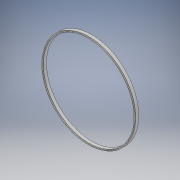
# Autodesk Inventor part: 뚜겅
Saved by Autodesk Inventor 2019.5 (Build 235369000, 369)
## iProperties
Created: 2021-07-28
Part Number: 뚜겅
Material: 일반
Document SubType Name: Modeling
Designer: msj19
Density: 1 g/cm^3
Appearance: 기본값
Author: msj19
Autodesk Inventor part; units mm, degrees
ref_plane "우측면도" through (0, 0, 0) normal (1, 0, 0) x (0, 1, 0)
ref_plane "평면도" through (0, 0, 0) normal (0, 1, 0) x (-1, 0, 0)
ref_plane "정면도" through (0, 0, 0) normal (0, 0, 1) x (1, 0, 0)
sketch "스케치1" plane through (0, 0, 0) normal (0, 0, 1) x (1, 0, 0)
  circle A0 centre (0, 0) radius 10
  circle A1 centre (0, 0) radius 155
  circle A2 centre (0, 0) radius 150
  line L0 (-100, -100) -> (100, -100)
  line L1 (100, -100) -> (100, 100)
  line L2 (100, 100) -> (-100, 100)
  line L3 (-100, 100) -> (-100, -100)
  line L4 (-100, -100) -> (100, 100) construction
  line L5 (100, -100) -> (-100, 100) construction
  point P0 (-92, -32.0118)
  dimension "d0" = 5
  dimension "d9" = 97.4103
  dimension "d10" = 200
  dimension "d11" = 200
  constraints: 12 end point, 3 centre point, 2 midpoint, 2 parallel, 1 coincident, 1 horizontal, 1 perpendicular
  measures "d0" radial gap between concentric circles of A1 A2
  measures "d9" distance of point (0, 0) point (-92, -32.012)
  measures "d10" distance of L2.end L1.end
  measures "d11" distance of L1.end L0.end
extrude "돌출1" add sketch "스케치1" along normal blind 10 contours A1
sketch "스케치2" plane through (0, 0, 10) normal (0, 0, 1) x (1, 0, 0)
  circle A0 centre (0, 0) radius 10
  circle A1 centre (0, 0) radius 150
  circle A2 centre (0, 0) radius 155
  circle A3 centre (0, 0) radius 151.6
  circle A4 centre (0, 0) radius 153.4
  point P0 (-92, -32.0118)
  dimension "d3" = 1.6
  dimension "d4" = 1.6
  constraints: 5 centre point, 2 coincident
  measures "d3" radial gap between concentric circles of A1 A3
  measures "d4" radial gap between concentric circles of A2 A4
extrude "돌출2" add sketch "스케치2" along normal blind 2.4 contours A4
